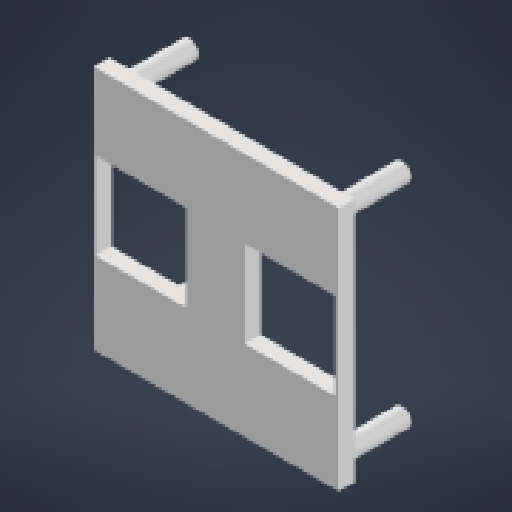
# Autodesk Inventor part: backplate
Saved by Autodesk Inventor 2024 (Build 280153000, 153)
## iProperties
Created: 2026-04-07
Part Number: backplate
Material: Generic
Document SubType Name: Modeling
Designer: schar
Density: 1 g/cm^3
Appearance: Default
Author: schar
Autodesk Inventor part; units mm, degrees
ref_plane "YZ Plane" through (0, 0, 0) normal (1, 0, 0) x (0, 1, 0)
ref_plane "XZ Plane" through (0, 0, 0) normal (0, 1, 0) x (-1, 0, 0)
ref_plane "XY Plane" through (0, 0, 0) normal (0, 0, 1) x (1, 0, 0)
sketch "Sketch1" plane through (0, 0, 0) normal (0, 0, 1) x (1, 0, 0)
  circle A0 centre (-102.5, -70) radius 1.1 projected
  circle A1 centre (-102.5, -70) radius 1.75
  line L0 (-99.4205, -113.1) -> (-99.4205, -66.9) projected
  line L1 (-145.5795, -113.1) -> (-99.4205, -113.1) projected
  line L2 (-145.5795, -66.9) -> (-145.5795, -113.1) projected
  line L3 (-99.4205, -66.9) -> (-145.5795, -66.9) projected
  line L4 (-97.5, -65) -> (-97.5, -115) projected
  line L5 (-147.5, -65) -> (-97.5, -65) projected
  line L6 (-147.5, -115) -> (-147.5, -65) projected
  line L7 (-97.5, -115) -> (-147.5, -115) projected
  line L8 (-122.5, -66.9) -> (-122.5, -113.1)
  line L9 (-145.5795, -90) -> (-99.4205, -90)
  circle A2 centre (-102.5, -70) radius 1.1
  circle A3 centre (-142.5, -70) radius 1.1
  circle A4 centre (-142.5, -70) radius 1.75
  circle A5 centre (-142.5, -110) radius 1.1
  circle A6 centre (-142.5, -110) radius 1.75
  circle A7 centre (-102.5, -110) radius 1.1
  circle A8 centre (-102.5, -110) radius 1.75
  point P0 (0, 0)
  point P1 (-122.5, -90)
  dimension "d0" = 3.5
  dimension "d3" = 360
  constraints: 8 centre point, 5 coincident, 5 midpoint, 4 end point, 1 concentric, 17 other
  measures "d0" diameter of A1
extrude "Extrusion1" add sketch "Sketch1" along normal blind 12 contours A1 | A4 | A6 | A8
sketch "Sketch2" plane through (-142.5, -70, 12) normal (0, 0, 1) x (1, 0, 0)
  line L0 (14.15, -26.93) -> (14.15, -11.83) projected
  line L1 (13.7, -11.38) -> (-2.1, -11.38) projected
  line L2 (-2.1, -27.38) -> (13.7, -27.38) projected
  line L3 (-2.55, -21.895) -> (-2.55, -16.865) projected
  line L4 (42.25, -17.215) -> (42.25, -22.245) projected
  line L5 (41.8, -11.73) -> (26, -11.73) projected
  line L6 (25.55, -12.18) -> (25.55, -27.28) projected
  line L7 (26, -27.73) -> (41.8, -27.73) projected
  line L8 (42.25, -19.73) -> (42.25, -27.73)
  line L9 (42.25, -27.73) -> (33.9, -27.73)
  line L10 (25.4, -11.58) -> (42.4, -11.58)
  line L11 (42.4, -11.58) -> (42.4, -27.88)
  line L12 (42.4, -27.88) -> (25.4, -27.88)
  line L13 (25.4, -27.88) -> (25.4, -11.58)
  line L14 (25.4, -11.58) -> (42.4, -27.88) construction
  line L15 (42.4, -11.58) -> (25.4, -27.88) construction
  line L16 (5.8, -27.38) -> (5.8, -19.38)
  line L17 (5.8, -19.38) -> (-2.55, -19.38)
  line L18 (-2.7, -11.23) -> (14.3, -11.23)
  line L19 (14.3, -11.23) -> (14.3, -27.53)
  line L20 (14.3, -27.53) -> (-2.7, -27.53)
  line L21 (-2.7, -27.53) -> (-2.7, -11.23)
  line L22 (-2.7, -11.23) -> (14.3, -27.53) construction
  line L23 (14.3, -11.23) -> (-2.7, -27.53) construction
  line L24 (-3.0795, -43.1) -> (43.0795, -43.1) projected
  line L25 (-3.0795, 3.1) -> (-3.0795, -43.1) projected
  line L26 (43.0795, -43.1) -> (43.0795, 3.1) projected
  line L27 (43.0795, 3.1) -> (-3.0795, 3.1) projected
  line L28 (-3.0795, -43.1) -> (43.0795, -43.1)
  line L29 (43.0795, -43.1) -> (43.0795, 3.1)
  line L30 (43.0795, 3.1) -> (-3.0795, 3.1)
  line L31 (-3.0795, 3.1) -> (-3.0795, -43.1)
  point P0 (142.5, 70)
  point P1 (33.9, -19.73)
  dimension "d7" = 17
  dimension "d8" = 16.3
  dimension "d9" = 17
  dimension "d10" = 16.3
  constraints: 40 end point, 8 midpoint, 6 parallel, 3 horizontal, 3 perpendicular, 2 vertical
  measures "d7" distance of L11.end L12.end
  measures "d8" distance of L10.end L11.end
  measures "d9" distance of L19.end L20.end
  measures "d10" distance of L18.end L19.end
extrude "Extrusion2" add sketch "Sketch2" along normal blind 3
sketch "Sketch3" plane through (-142.5, -70, 15) normal (0, 0, 1) x (1, 0, 0)
  line L0 (3.8499, -5.182) -> (7.7501, -5.182) construction
  line L1 (7.7501, -5.182) -> (7.7501, -8.23) construction
  line L2 (7.7501, -8.23) -> (3.8499, -8.23) construction
  line L3 (3.8499, -8.23) -> (3.8499, -5.182) construction
  line L4 (30.547, -5.4036) -> (37.253, -5.4036) construction
  line L5 (37.253, -5.4036) -> (37.253, -8.58) construction
  line L6 (37.253, -8.58) -> (30.547, -8.58) construction
  line L7 (30.547, -8.58) -> (30.547, -5.4036) construction
  line L8 (-2.7, -11.23) -> (14.3, -11.23) projected
  line L9 (5.8, -11.23) -> (5.8, -8.23)
  line L10 (3.8499, -8.23) -> (7.7501, -8.23)
  line L11 (25.4, -11.58) -> (42.4, -11.58) projected
  line L12 (33.9, -11.58) -> (33.9, -8.58)
  line L13 (30.547, -8.58) -> (37.253, -8.58)
  line L14 (5.2208, -8.23) -> (4.0401, -8.23)
  line L15 (4.0401, -8.23) -> (4.0401, -7.9188)
  line L16 (4.0401, -7.9188) -> (4.4279, -7.9188)
  line L17 (4.4279, -7.9188) -> (4.4279, -5.4932)
  line L18 (4.4279, -5.4932) -> (4.0401, -5.4932)
  line L19 (4.0401, -5.4932) -> (4.0401, -5.182)
  line L20 (4.0401, -5.182) -> (5.2208, -5.182)
  line L21 (5.2208, -5.182) -> (5.2208, -5.4932)
  line L22 (5.2208, -5.4932) -> (4.833, -5.4932)
  line L23 (4.833, -5.4932) -> (4.833, -7.9188)
  line L24 (4.833, -7.9188) -> (5.2208, -7.9188)
  line L25 (5.2208, -7.9188) -> (5.2208, -8.23)
  line L26 (7.4883, -8.23) -> (7.1029, -8.23)
  line L27 (7.1029, -8.23) -> (7.1029, -6.9258)
  spline S0 degree 2 poles (7.1029, -6.9258) (7.1029, -6.7678) (7.0733, -6.496) (7.0288, -6.4145) knots 0 0 0 1 2 2 2
  spline S1 degree 2 poles (7.0288, -6.4145) (6.9819, -6.3281) (6.8139, -6.2441) (6.6707, -6.2441) knots 0 0 0 1 2 2 2
  spline S2 degree 2 poles (6.6707, -6.2441) (6.5274, -6.2441) (6.2236, -6.3972) (6.0779, -6.5207) knots 0 0 0 1 2 2 2
  line L28 (6.0779, -6.5207) -> (6.0779, -8.23)
  line L29 (6.0779, -8.23) -> (5.6926, -8.23)
  line L30 (5.6926, -8.23) -> (5.6926, -5.9428)
  line L31 (5.6926, -5.9428) -> (6.0779, -5.9428)
  line L32 (6.0779, -5.9428) -> (6.0779, -6.1972)
  spline S3 degree 2 poles (6.0779, -6.1972) (6.2508, -6.0416) (6.5842, -5.8785) (6.772, -5.8785) knots 0 0 0 1 2 2 2
  spline S4 degree 2 poles (6.772, -5.8785) (7.1079, -5.8785) (7.4883, -6.3231) (7.4883, -6.7455) knots 0 0 0 1 2 2 2
  line L33 (7.4883, -6.7455) -> (7.4883, -8.23)
  spline S5 degree 2 poles (33.012, -5.8161) (33.1849, -6.0186) (33.3776, -6.6114) (33.3776, -6.9918) knots 0 0 0 1 2 2 2
  spline S6 degree 2 poles (33.3776, -6.9918) (33.3776, -7.3623) (33.1899, -7.9625) (33.012, -8.165) knots 0 0 0 1 2 2 2
  spline S7 degree 2 poles (33.012, -8.165) (32.8243, -8.3775) (32.3278, -8.58) (32.029, -8.58) knots 0 0 0 1 2 2 2
  spline S8 degree 2 poles (32.029, -8.58) (31.7202, -8.58) (31.2262, -8.37) (31.0459, -8.165) knots 0 0 0 1 2 2 2
  spline S9 degree 2 poles (31.0459, -8.165) (30.8705, -7.9625) (30.6828, -7.3672) (30.6828, -6.9918) knots 0 0 0 1 2 2 2
  spline S10 degree 2 poles (30.6828, -6.9918) (30.6828, -6.6089) (30.873, -6.026) (31.0484, -5.8161) knots 0 0 0 1 2 2 2
  spline S11 degree 2 poles (31.0484, -5.8161) (31.2262, -5.6135) (31.7227, -5.4036) (32.029, -5.4036) knots 0 0 0 1 2 2 2
  spline S12 degree 2 poles (32.029, -5.4036) (32.3402, -5.4036) (32.8391, -5.6209) (33.012, -5.8161) knots 0 0 0 1 2 2 2
  spline S13 degree 2 poles (32.9552, -6.9918) (32.9552, -6.6904) (32.8243, -6.2236) (32.7057, -6.0705) knots 0 0 0 1 2 2 2
  spline S14 degree 2 poles (32.7057, -6.0705) (32.5847, -5.9124) (32.2439, -5.7543) (32.0314, -5.7543) knots 0 0 0 1 2 2 2
  spline S15 degree 2 poles (32.0314, -5.7543) (31.8116, -5.7543) (31.4806, -5.9074) (31.3546, -6.0705) knots 0 0 0 1 2 2 2
  spline S16 degree 2 poles (31.3546, -6.0705) (31.2336, -6.2261) (31.1052, -6.6954) (31.1052, -6.9918) knots 0 0 0 1 2 2 2
  spline S17 degree 2 poles (31.1052, -6.9918) (31.1052, -7.592) (31.6091, -8.2293) (32.0314, -8.2293) knots 0 0 0 1 2 2 2
  spline S18 degree 2 poles (32.0314, -8.2293) (32.4538, -8.2293) (32.9552, -7.592) (32.9552, -6.9918) knots 0 0 0 1 2 2 2
  line L34 (35.571, -8.5158) -> (35.1856, -8.5158)
  line L35 (35.1856, -8.5158) -> (35.1856, -8.2638)
  spline S19 degree 2 poles (35.1856, -8.2638) (35.0078, -8.4194) (34.6892, -8.58) (34.4916, -8.58) knots 0 0 0 1 2 2 2
  spline S20 degree 2 poles (34.4916, -8.58) (34.3434, -8.58) (34.0791, -8.4812) (33.9827, -8.375) knots 0 0 0 1 2 2 2
  spline S21 degree 2 poles (33.9827, -8.375) (33.8839, -8.2688) (33.7753, -7.9452) (33.7753, -7.713) knots 0 0 0 1 2 2 2
  line L36 (33.7753, -7.713) -> (33.7753, -6.2285)
  line L37 (33.7753, -6.2285) -> (34.1606, -6.2285)
  line L38 (34.1606, -6.2285) -> (34.1606, -7.5327)
  spline S22 degree 2 poles (34.1606, -7.5327) (34.1606, -7.7155) (34.1878, -7.9551) (34.2347, -8.044) knots 0 0 0 1 2 2 2
  spline S23 degree 2 poles (34.2347, -8.044) (34.2816, -8.1329) (34.4422, -8.2144) (34.5928, -8.2144) knots 0 0 0 1 2 2 2
  spline S24 degree 2 poles (34.5928, -8.2144) (34.7336, -8.2144) (35.0523, -8.0539) (35.1856, -7.9378) knots 0 0 0 1 2 2 2
  line L39 (35.1856, -7.9378) -> (35.1856, -6.2285)
  line L40 (35.1856, -6.2285) -> (35.571, -6.2285)
  line L41 (35.571, -6.2285) -> (35.571, -8.5158)
  spline S25 degree 2 poles (36.8208, -8.5602) (36.5071, -8.5602) (36.1539, -8.2021) (36.1539, -7.8143) knots 0 0 0 1 2 2 2
  line L42 (36.1539, -7.8143) -> (36.1539, -6.5472)
  line L43 (36.1539, -6.5472) -> (35.8945, -6.5472)
  line L44 (35.8945, -6.5472) -> (35.8945, -6.2285)
  line L45 (35.8945, -6.2285) -> (36.1539, -6.2285)
  line L46 (36.1539, -6.2285) -> (36.1539, -5.5715)
  line L47 (36.1539, -5.5715) -> (36.5392, -5.5715)
  line L48 (36.5392, -5.5715) -> (36.5392, -6.2285)
  line L49 (36.5392, -6.2285) -> (37.2481, -6.2285)
  line L50 (37.2481, -6.2285) -> (37.2481, -6.5472)
  line L51 (37.2481, -6.5472) -> (36.5392, -6.5472)
  line L52 (36.5392, -6.5472) -> (36.5392, -7.6365)
  spline S26 degree 2 poles (36.5392, -7.6365) (36.5392, -7.8094) (36.5516, -7.9995) (36.5936, -8.0811) knots 0 0 0 1 2 2 2
  spline S27 degree 2 poles (36.5936, -8.0811) (36.6281, -8.1527) (36.7837, -8.2243) (36.9171, -8.2243) knots 0 0 0 1 2 2 2
  spline S28 degree 2 poles (36.9171, -8.2243) (37.011, -8.2243) (37.1864, -8.1675) (37.2259, -8.1502) knots 0 0 0 1 2 2 2
  line L53 (37.2259, -8.1502) -> (37.2481, -8.1502)
  line L54 (37.2481, -8.1502) -> (37.2481, -8.496)
  spline S29 degree 2 poles (37.2481, -8.496) (37.1394, -8.5257) (36.9171, -8.5602) (36.8208, -8.5602) knots 0 0 0 1 2 2 2
  point P0 (142.5, 70)
  dimension "d13" = 3
  dimension "d14" = 3
  constraints: 8 end point, 4 midpoint, 2 collinear, 2 vertical, 4 other
  measures "d13" distance of L9.end L9.start
  measures "d14" distance of L12.end L12.start
extrude "Extrusion3" cut sketch "Sketch3" against normal blind 0.5 contours L15 L16 L17 L18 L19 L20 L21 L22 L23 L24 L25 L10 | L30 L31 L32 S3 S4 L33 L10 L27 S0 S1 S2 L28 | S5 S6 S7 S8 S9 S10 S11 S12 | L34 L35 S19 S20 S21 L36 L37 L38 S22 S23 S24 L39 L40 L41 | S25 L42 L43 L44 L45 L46 L47 L48 L49 L50 L51 L52 S26 S27 S28 L53 L54 S29
sketch "Sketch4" plane through (-145.5795, -113.1, 12) normal (-1, 0, 0) x (0, 0, 1)
  line L0 (0, 46.2) -> (0, 0) projected
  line L1 (3, 46.2) -> (-13.51, 46.2) projected
  line L2 (3, -1.9) -> (3, 48.1) projected
  line L3 (3, 0) -> (-13.51, 0) projected
  point P0 (-12, 113.1)
extrude "Extrusion4" cut sketch "Sketch4" against normal blind 0.3
sketch "Sketch5" plane through (-99.4205, -66.9, 15) normal (0, 1, 0) x (1, 0, 0)
  line L0 (0, 3) -> (-45.859, 3) projected
  line L1 (0, 16.51) -> (0, 0) projected
  line L2 (-48.0795, 0) -> (1.9205, 0) projected
  line L3 (-45.859, 3) -> (-45.859, 0) projected
  point P0 (99.4205, 15)
extrude "Extrusion5" cut sketch "Sketch5" against normal blind 0.3
sketch "Sketch6" plane through (-99.4205, -113.1, 15) normal (1, 0, 0) x (0, 0, -1)
  line L0 (3, 0) -> (3, 45.9) projected
  line L1 (0, 0) -> (16.51, 0) projected
  line L2 (0, 48.1) -> (0, -1.9) projected
  line L3 (3, 45.9) -> (0, 45.9) projected
  point P0 (15, 113.1)
extrude "Extrusion6" cut sketch "Sketch6" against normal blind 0.3
sketch "Sketch7" plane through (-145.2795, -113.1, 12) normal (0, -1, 0) x (1, 0, 0)
  line L0 (0, 3) -> (0, 0) projected
  line L1 (0, 0) -> (45.559, 0) projected
  line L2 (47.7795, 3) -> (-2.2205, 3) projected
  line L3 (45.559, 0) -> (45.559, 3) projected
  point P0 (145.2795, -12)
extrude "Extrusion7" cut sketch "Sketch7" against normal blind 0.3
body "Solid1"
